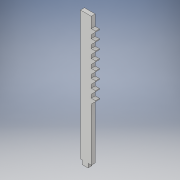
# Autodesk Inventor part: graduated_foot_02
Saved by Autodesk Inventor 2019.4 (Build 234330000, 330)
## iProperties
Created: 2019-12-18
Part Number: graduated_foot_02
Material: Generic
Document SubType Name: Modeling
Designer: fabfarm
Density: 1 g/cm^3
Appearance: Default
Author: fabfarm
Autodesk Inventor part; units mm, degrees
ref_plane "YZ Plane" through (0, 0, 0) normal (1, 0, 0) x (0, 1, 0)
ref_plane "XZ Plane" through (0, 0, 0) normal (0, 1, 0) x (-1, 0, 0)
ref_plane "XY Plane" through (0, 0, 0) normal (0, 0, 1) x (1, 0, 0)
sketch "Sketch1" plane through (0, 0, 0) normal (0, 0, 1) x (1, 0, 0)
  line L0 (0, 0) -> (50, 0)
  line L1 (50, 0) -> (50, 600)
  line L2 (50, 600) -> (0, 600)
  line L3 (0, 600) -> (0, 0)
  dimension "d0" = 600
  dimension "d1" = 50
  constraints: 8 end point, 2 parallel, 1 horizontal, 1 perpendicular
  measures "d0" distance of L0.end L1.end
  measures "d1" distance of L0.start L0.end
extrude "Extrusion1" add sketch "Sketch1" along normal blind 18.55
sketch "Sketch2" plane through (0, 0, 18.55) normal (0, 0, 1) x (1, 0, 0)
  line L0 (50, 0) -> (50, 600) projected
  line L1 (50, 550) -> (70, 550)
  line L2 (70, 550) -> (70, 546)
  line L3 (70, 546) -> (50, 526)
  line L4 (50, 600) -> (0, 600) projected
  line L5 (0, 0) -> (50, 0) projected
  line L6 (10, 0) -> (35, 0)
  line L7 (35, 0) -> (35, -18.55)
  line L8 (35, -18.55) -> (10, -18.55)
  line L9 (10, -18.55) -> (10, 0)
  line L10 (0, 600) -> (0, 0) projected
  line L11 (50, 550) -> (50, 526)
  line L12 (50, 510) -> (70, 510)
  line L13 (70, 510) -> (70, 506)
  line L14 (70, 506) -> (50, 486)
  line L15 (50, 510) -> (50, 486)
  line L16 (50, 470) -> (70, 470)
  line L17 (70, 470) -> (70, 466)
  line L18 (70, 466) -> (50, 446)
  line L19 (50, 470) -> (50, 446)
  line L20 (50, 430) -> (70, 430)
  line L21 (70, 430) -> (70, 426)
  line L22 (70, 426) -> (50, 406)
  line L23 (50, 430) -> (50, 406)
  line L24 (50, 390) -> (70, 390)
  line L25 (70, 390) -> (70, 386)
  line L26 (70, 386) -> (50, 366)
  line L27 (50, 390) -> (50, 366)
  line L28 (50, 350) -> (70, 350)
  line L29 (70, 350) -> (70, 346)
  line L30 (70, 346) -> (50, 326)
  line L31 (50, 350) -> (50, 326)
  line L32 (50, 310) -> (70, 310)
  line L33 (70, 310) -> (70, 306)
  line L34 (70, 306) -> (50, 286)
  line L35 (50, 310) -> (50, 286)
  line L36 (50, 270) -> (70, 270)
  line L37 (70, 270) -> (70, 266)
  line L38 (70, 266) -> (50, 246)
  line L39 (50, 270) -> (50, 246)
  dimension "d4" = 50
  dimension "d5" = 4
  dimension "d6" = 20
  dimension "d7" = 45
  dimension "d15" = 15
  dimension "d16" = 25
  dimension "d17" = 10
  dimension "d18" = 18.55
  dimension "d21" = 40
  constraints: 72 end point, 3 point on line, 2 horizontal, 2 parallel, 2 perpendicular, 1 collinear, 1 vertical, 56 other
  measures "d4" distance between parallel lines of L4 L1
  measures "d5" distance of L1.end L2.end
  measures "d6" distance of L1.start L1.end
  measures "d7" angle of L0 L3
  measures "d15" distance between parallel lines of L0 L7
  measures "d16" distance of L7.end L8.end
  measures "d17" distance between parallel lines of L10 L9
  measures "d18" distance of L6.end L7.end
  measures "d21" distance of L1.start L12.start
extrude "Extrusion2" add sketch "Sketch2" against normal blind 18.55 contours L0 L36 L37 L38 | L7 L8 L9 L5 | L0 L32 L33 L34 | L0 L28 L29 L30 | L1 L2 L3 L0 | L0 L24 L25 L26 | L12 L13 L14 L0 | L0 L20 L21 L22 | L16 L17 L18 L0
body "Solid1"
